Autodesk Inventor part; units mm, degrees
(part 2 of 6)
  line L925 (26.7951, -12.8841) -> (26.6059, -12.8584)
  line L926 (26.6059, -12.8584) -> (26.4288, -12.8305)
  line L927 (26.4288, -12.8305) -> (26.0833, -12.7672)
  line L928 (26.0833, -12.7672) -> (26.0365, -12.7656)
  line L929 (26.0365, -12.7656) -> (26.0012, -12.7712)
  line L930 (26.0012, -12.7712) -> (25.9777, -12.7837)
  line L931 (25.9777, -12.7837) -> (25.968, -12.7973)
  line L932 (25.968, -12.7973) -> (25.7946, -13.143)
  line L933 (25.7946, -13.143) -> (25.6168, -13.4865)
  line L934 (25.6168, -13.4865) -> (25.6116, -13.5023)
  line L935 (25.6116, -13.5023) -> (25.6153, -13.5287)
  line L936 (25.6153, -13.5287) -> (25.6314, -13.5605)
  line L937 (25.6314, -13.5605) -> (25.6603, -13.5974)
  line L938 (25.6603, -13.5974) -> (25.9146, -13.8398)
  line L939 (25.9146, -13.8398) -> (26.0412, -13.9666)
  line L940 (26.0412, -13.9666) -> (26.1732, -14.1046)
  line L941 (26.1732, -14.1046) -> (26.312, -14.2558)
  line L942 (26.312, -14.2558) -> (26.455, -14.4184)
  line L943 (26.455, -14.4184) -> (26.602, -14.5927)
  line L944 (26.602, -14.5927) -> (26.7541, -14.7808)
  line L945 (26.7541, -14.7808) -> (26.9091, -14.9811)
  line L946 (26.9091, -14.9811) -> (27.041, -15.1586)
  arc A24 (26.6482, -15.8389) -> (27.041, -15.1586) centre (0, 0) ccw
  line L947 (26.6482, -15.8389) -> (26.4285, -15.8134)
  line L948 (26.4285, -15.8134) -> (26.1776, -15.7793)
  line L949 (26.1776, -15.7793) -> (25.9387, -15.7417)
  line L950 (25.9387, -15.7417) -> (25.7142, -15.7015)
  line L951 (25.7142, -15.7015) -> (25.5018, -15.6589)
  line L952 (25.5018, -15.6589) -> (25.3015, -15.6144)
  line L953 (25.3015, -15.6144) -> (25.1161, -15.569)
  line L954 (25.1161, -15.569) -> (24.9429, -15.5228)
  line L955 (24.9429, -15.5228) -> (24.6058, -15.4237)
  line L956 (24.6058, -15.4237) -> (24.5595, -15.4172)
  line L957 (24.5595, -15.4172) -> (24.5238, -15.4191)
  line L958 (24.5238, -15.4191) -> (24.4991, -15.4291)
  line L959 (24.4991, -15.4291) -> (24.488, -15.4416)
  line L960 (24.488, -15.4416) -> (24.2795, -15.7673)
  line L961 (24.2795, -15.7673) -> (24.0668, -16.0903)
  line L962 (24.0668, -16.0903) -> (24.0599, -16.1055)
  line L963 (24.0599, -16.1055) -> (24.0608, -16.1321)
  line L964 (24.0608, -16.1321) -> (24.0735, -16.1655)
  line L965 (24.0735, -16.1655) -> (24.0984, -16.2052)
  line L966 (24.0984, -16.2052) -> (24.326, -16.4728)
  line L967 (24.326, -16.4728) -> (24.4386, -16.6122)
  line L968 (24.4386, -16.6122) -> (24.5555, -16.7632)
  line L969 (24.5555, -16.7632) -> (24.6777, -16.928)
  line L970 (24.6777, -16.928) -> (24.8029, -17.1047)
  line L971 (24.8029, -17.1047) -> (24.931, -17.2934)
  line L972 (24.931, -17.2934) -> (25.0625, -17.4964)
  line L973 (25.0625, -17.4964) -> (25.1957, -17.7118)
  line L974 (25.1957, -17.7118) -> (25.3084, -17.9021)
  arc A25 (24.8466, -18.5377) -> (25.3084, -17.9021) centre (0, 0) ccw
  line L975 (24.8466, -18.5377) -> (24.6308, -18.4893)
  line L976 (24.6308, -18.4893) -> (24.3848, -18.4292)
  line L977 (24.3848, -18.4292) -> (24.1511, -18.3668)
  line L978 (24.1511, -18.3668) -> (23.932, -18.3034)
  line L979 (23.932, -18.3034) -> (23.7253, -18.2388)
  line L980 (23.7253, -18.2388) -> (23.5308, -18.1736)
  line L981 (23.5308, -18.1736) -> (23.3511, -18.1091)
  line L982 (23.3511, -18.1091) -> (23.1837, -18.045)
  line L983 (23.1837, -18.045) -> (22.8588, -17.9112)
  line L984 (22.8588, -17.9112) -> (22.8134, -17.8999)
  line L985 (22.8134, -17.8999) -> (22.7777, -17.8981)
  line L986 (22.7777, -17.8981) -> (22.7521, -17.9055)
  line L987 (22.7521, -17.9055) -> (22.7398, -17.9167)
  line L988 (22.7398, -17.9167) -> (22.4984, -18.2188)
  line L989 (22.4984, -18.2188) -> (22.2531, -18.5178)
  line L990 (22.2531, -18.5178) -> (22.2446, -18.5322)
  line L991 (22.2446, -18.5322) -> (22.2427, -18.5587)
  line L992 (22.2427, -18.5587) -> (22.2519, -18.5933)
  line L993 (22.2519, -18.5933) -> (22.2724, -18.6353)
  line L994 (22.2724, -18.6353) -> (22.4708, -18.9253)
  line L995 (22.4708, -18.9253) -> (22.5683, -19.0757)
  line L996 (22.5683, -19.0757) -> (22.6688, -19.2381)
  line L997 (22.6688, -19.2381) -> (22.773, -19.4148)
  line L998 (22.773, -19.4148) -> (22.8791, -19.6036)
  line L999 (22.8791, -19.6036) -> (22.9867, -19.8047)
  line L1000 (22.9867, -19.8047) -> (23.0963, -20.0203)
  line L1001 (23.0963, -20.0203) -> (23.2063, -20.2484)
  line L1002 (23.2063, -20.2484) -> (23.2985, -20.4495)
  arc A26 (22.7728, -21.0333) -> (23.2985, -20.4495) centre (0, 0) ccw
  line L1003 (22.7728, -21.0333) -> (22.5632, -20.9626)
  line L1004 (22.5632, -20.9626) -> (22.3249, -20.8771)
  line L1005 (22.3249, -20.8771) -> (22.099, -20.7906)
  line L1006 (22.099, -20.7906) -> (21.8877, -20.7047)
  line L1007 (21.8877, -20.7047) -> (21.6889, -20.6189)
  line L1008 (21.6889, -20.6189) -> (21.5022, -20.5336)
  line L1009 (21.5022, -20.5336) -> (21.3302, -20.4507)
  line L1010 (21.3302, -20.4507) -> (21.1705, -20.3695)
  line L1011 (21.1705, -20.3695) -> (20.8614, -20.2025)
  line L1012 (20.8614, -20.2025) -> (20.8174, -20.1865)
  line L1013 (20.8174, -20.1865) -> (20.7821, -20.181)
  line L1014 (20.7821, -20.181) -> (20.7559, -20.1856)
  line L1015 (20.7559, -20.1856) -> (20.7424, -20.1955)
  line L1016 (20.7424, -20.1955) -> (20.4707, -20.4707)
  line L1017 (20.4707, -20.4707) -> (20.1955, -20.7424)
  line L1018 (20.1955, -20.7424) -> (20.1856, -20.7559)
  line L1019 (20.1856, -20.7559) -> (20.181, -20.7821)
  line L1020 (20.181, -20.7821) -> (20.1865, -20.8174)
  line L1021 (20.1865, -20.8174) -> (20.2025, -20.8614)
  line L1022 (20.2025, -20.8614) -> (20.3695, -21.1705)
  line L1023 (20.3695, -21.1705) -> (20.4507, -21.3302)
  line L1024 (20.4507, -21.3302) -> (20.5336, -21.5022)
  line L1025 (20.5336, -21.5022) -> (20.6189, -21.6889)
  line L1026 (20.6189, -21.6889) -> (20.7047, -21.8877)
  line L1027 (20.7047, -21.8877) -> (20.7906, -22.099)
  line L1028 (20.7906, -22.099) -> (20.8771, -22.3249)
  line L1029 (20.8771, -22.3249) -> (20.9626, -22.5632)
  line L1030 (20.9626, -22.5632) -> (21.0333, -22.7728)
  arc A27 (20.4495, -23.2985) -> (21.0333, -22.7728) centre (0, 0) ccw
  line L1031 (20.4495, -23.2985) -> (20.2484, -23.2063)
  line L1032 (20.2484, -23.2063) -> (20.0203, -23.0963)
  line L1033 (20.0203, -23.0963) -> (19.8047, -22.9867)
  line L1034 (19.8047, -22.9867) -> (19.6036, -22.8791)
  line L1035 (19.6036, -22.8791) -> (19.4148, -22.773)
  line L1036 (19.4148, -22.773) -> (19.2381, -22.6688)
  line L1037 (19.2381, -22.6688) -> (19.0757, -22.5683)
  line L1038 (19.0757, -22.5683) -> (18.9253, -22.4708)
  line L1039 (18.9253, -22.4708) -> (18.6353, -22.2724)
  line L1040 (18.6353, -22.2724) -> (18.5933, -22.2519)
  line L1041 (18.5933, -22.2519) -> (18.5587, -22.2427)
  line L1042 (18.5587, -22.2427) -> (18.5322, -22.2446)
  line L1043 (18.5322, -22.2446) -> (18.5178, -22.2531)
  line L1044 (18.5178, -22.2531) -> (18.2188, -22.4984)
  line L1045 (18.2188, -22.4984) -> (17.9167, -22.7398)
  line L1046 (17.9167, -22.7398) -> (17.9055, -22.7521)
  line L1047 (17.9055, -22.7521) -> (17.8981, -22.7777)
  line L1048 (17.8981, -22.7777) -> (17.8999, -22.8134)
  line L1049 (17.8999, -22.8134) -> (17.9112, -22.8588)
  line L1050 (17.9112, -22.8588) -> (18.045, -23.1837)
  line L1051 (18.045, -23.1837) -> (18.1091, -23.3511)
  line L1052 (18.1091, -23.3511) -> (18.1736, -23.5308)
  line L1053 (18.1736, -23.5308) -> (18.2388, -23.7253)
  line L1054 (18.2388, -23.7253) -> (18.3034, -23.932)
  line L1055 (18.3034, -23.932) -> (18.3668, -24.1511)
  line L1056 (18.3668, -24.1511) -> (18.4292, -24.3848)
  line L1057 (18.4292, -24.3848) -> (18.4893, -24.6308)
  line L1058 (18.4893, -24.6308) -> (18.5377, -24.8466)
  arc A28 (17.9021, -25.3084) -> (18.5377, -24.8466) centre (0, 0) ccw
  line L1059 (17.9021, -25.3084) -> (17.7118, -25.1957)
  line L1060 (17.7118, -25.1957) -> (17.4964, -25.0625)
  line L1061 (17.4964, -25.0625) -> (17.2934, -24.931)
  line L1062 (17.2934, -24.931) -> (17.1047, -24.8029)
  line L1063 (17.1047, -24.8029) -> (16.928, -24.6777)
  line L1064 (16.928, -24.6777) -> (16.7632, -24.5555)
  line L1065 (16.7632, -24.5555) -> (16.6122, -24.4386)
  line L1066 (16.6122, -24.4386) -> (16.4728, -24.326)
  line L1067 (16.4728, -24.326) -> (16.2052, -24.0984)
  line L1068 (16.2052, -24.0984) -> (16.1655, -24.0735)
  line L1069 (16.1655, -24.0735) -> (16.1321, -24.0608)
  line L1070 (16.1321, -24.0608) -> (16.1055, -24.0599)
  line L1071 (16.1055, -24.0599) -> (16.0903, -24.0668)
  line L1072 (16.0903, -24.0668) -> (15.7673, -24.2795)
  line L1073 (15.7673, -24.2795) -> (15.4416, -24.488)
  line L1074 (15.4416, -24.488) -> (15.4291, -24.4991)
  line L1075 (15.4291, -24.4991) -> (15.4191, -24.5238)
  line L1076 (15.4191, -24.5238) -> (15.4172, -24.5595)
  line L1077 (15.4172, -24.5595) -> (15.4237, -24.6058)
  line L1078 (15.4237, -24.6058) -> (15.5228, -24.9429)
  line L1079 (15.5228, -24.9429) -> (15.569, -25.1161)
  line L1080 (15.569, -25.1161) -> (15.6144, -25.3015)
  line L1081 (15.6144, -25.3015) -> (15.6589, -25.5018)
  line L1082 (15.6589, -25.5018) -> (15.7015, -25.7142)
  line L1083 (15.7015, -25.7142) -> (15.7417, -25.9387)
  line L1084 (15.7417, -25.9387) -> (15.7793, -26.1776)
  line L1085 (15.7793, -26.1776) -> (15.8134, -26.4285)
  line L1086 (15.8134, -26.4285) -> (15.8389, -26.6482)
  arc A29 (15.1586, -27.041) -> (15.8389, -26.6482) centre (0, 0) ccw
  line L1087 (15.1586, -27.041) -> (14.9811, -26.9091)
  line L1088 (14.9811, -26.9091) -> (14.7808, -26.7541)
  line L1089 (14.7808, -26.7541) -> (14.5927, -26.602)
  line L1090 (14.5927, -26.602) -> (14.4184, -26.455)
  line L1091 (14.4184, -26.455) -> (14.2558, -26.312)
  line L1092 (14.2558, -26.312) -> (14.1046, -26.1732)
  line L1093 (14.1046, -26.1732) -> (13.9666, -26.0412)
  line L1094 (13.9666, -26.0412) -> (13.8398, -25.9146)
  line L1095 (13.8398, -25.9146) -> (13.5974, -25.6603)
  line L1096 (13.5974, -25.6603) -> (13.5605, -25.6314)
  line L1097 (13.5605, -25.6314) -> (13.5287, -25.6153)
  line L1098 (13.5287, -25.6153) -> (13.5023, -25.6116)
  line L1099 (13.5023, -25.6116) -> (13.4865, -25.6168)
  line L1100 (13.4865, -25.6168) -> (13.143, -25.7946)
  line L1101 (13.143, -25.7946) -> (12.7973, -25.968)
  line L1102 (12.7973, -25.968) -> (12.7837, -25.9777)
  line L1103 (12.7837, -25.9777) -> (12.7712, -26.0012)
  line L1104 (12.7712, -26.0012) -> (12.7656, -26.0365)
  line L1105 (12.7656, -26.0365) -> (12.7672, -26.0833)
  line L1106 (12.7672, -26.0833) -> (12.8305, -26.4288)
  line L1107 (12.8305, -26.4288) -> (12.8584, -26.6059)
  line L1108 (12.8584, -26.6059) -> (12.8841, -26.7951)
  line L1109 (12.8841, -26.7951) -> (12.9075, -26.9989)
  line L1110 (12.9075, -26.9989) -> (12.9276, -27.2145)
  line L1111 (12.9276, -27.2145) -> (12.9441, -27.442)
  line L1112 (12.9441, -27.442) -> (12.9565, -27.6836)
  line L1113 (12.9565, -27.6836) -> (12.9642, -27.9367)
  line L1114 (12.9642, -27.9367) -> (12.9667, -28.1579)
  arc A30 (12.249, -28.4774) -> (12.9667, -28.1579) centre (0, 0) ccw
  line L1115 (12.249, -28.4774) -> (12.0862, -28.3276)
  line L1116 (12.0862, -28.3276) -> (11.9033, -28.1525)
  line L1117 (11.9033, -28.1525) -> (11.7321, -27.9817)
  line L1118 (11.7321, -27.9817) -> (11.5741, -27.8172)
  line L1119 (11.5741, -27.8172) -> (11.4273, -27.6579)
  line L1120 (11.4273, -27.6579) -> (11.2915, -27.5042)
  line L1121 (11.2915, -27.5042) -> (11.1681, -27.3584)
  line L1122 (11.1681, -27.3584) -> (11.0551, -27.2193)
  line L1123 (11.0551, -27.2193) -> (10.8407, -26.941)
  line L1124 (10.8407, -26.941) -> (10.807, -26.9085)
  line L1125 (10.807, -26.9085) -> (10.777, -26.8891)
  line L1126 (10.777, -26.8891) -> (10.7512, -26.8826)
  line L1127 (10.7512, -26.8826) -> (10.7349, -26.8862)
  line L1128 (10.7349, -26.8862) -> (10.3748, -27.0272)
  line L1129 (10.3748, -27.0272) -> (10.0128, -27.1634)
  line L1130 (10.0128, -27.1634) -> (9.9983, -27.1717)
  line L1131 (9.9983, -27.1717) -> (9.9834, -27.1937)
  line L1132 (9.9834, -27.1937) -> (9.9741, -27.2282)
  line L1133 (9.9741, -27.2282) -> (9.9708, -27.2749)
  line L1134 (9.9708, -27.2749) -> (9.9977, -27.6252)
  line L1135 (9.9977, -27.6252) -> (10.0069, -27.8042)
  line L1136 (10.0069, -27.8042) -> (10.0127, -27.995)
  line L1137 (10.0127, -27.995) -> (10.0146, -28.2002)
  line L1138 (10.0146, -28.2002) -> (10.0121, -28.4168)
  line L1139 (10.0121, -28.4168) -> (10.0047, -28.6447)
  line L1140 (10.0047, -28.6447) -> (9.9918, -28.8863)
  line L1141 (9.9918, -28.8863) -> (9.973, -29.1388)
  line L1142 (9.973, -29.1388) -> (9.9523, -29.359)
  arc A31 (9.2052, -29.6018) -> (9.9523, -29.359) centre (0, 0) ccw
  line L1143 (9.2052, -29.6018) -> (9.059, -29.4358)
  line L1144 (9.059, -29.4358) -> (8.8954, -29.2425)
  line L1145 (8.8954, -29.2425) -> (8.7429, -29.0547)
  line L1146 (8.7429, -29.0547) -> (8.603, -28.8746)
  line L1147 (8.603, -28.8746) -> (8.4737, -28.7009)
  line L1148 (8.4737, -28.7009) -> (8.3547, -28.5338)
  line L1149 (8.3547, -28.5338) -> (8.2472, -28.3759)
  line L1150 (8.2472, -28.3759) -> (8.1494, -28.2257)
  line L1151 (8.1494, -28.2257) -> (7.9652, -27.9266)
  line L1152 (7.9652, -27.9266) -> (7.9351, -27.8907)
  line L1153 (7.9351, -27.8907) -> (7.9073, -27.8683)
  line L1154 (7.9073, -27.8683) -> (7.8823, -27.8592)
  line L1155 (7.8823, -27.8592) -> (7.8657, -27.861)
  line L1156 (7.8657, -27.861) -> (7.4928, -27.9636)
  line L1157 (7.4928, -27.9636) -> (7.1186, -28.0612)
  line L1158 (7.1186, -28.0612) -> (7.1033, -28.0679)
  line L1159 (7.1033, -28.0679) -> (7.0862, -28.0883)
  line L1160 (7.0862, -28.0883) -> (7.0733, -28.1216)
  line L1161 (7.0733, -28.1216) -> (7.0652, -28.1677)
  line L1162 (7.0652, -28.1677) -> (7.0553, -28.5189)
  line L1163 (7.0553, -28.5189) -> (7.0457, -28.6979)
  line L1164 (7.0457, -28.6979) -> (7.0315, -28.8883)
  line L1165 (7.0315, -28.8883) -> (7.012, -29.0926)
  line L1166 (7.012, -29.0926) -> (6.9869, -29.3077)
  line L1167 (6.9869, -29.3077) -> (6.9557, -29.5336)
  line L1168 (6.9557, -29.5336) -> (6.9177, -29.7725)
  line L1169 (6.9177, -29.7725) -> (6.8726, -30.0216)
  line L1170 (6.8726, -30.0216) -> (6.829, -30.2385)
  arc A32 (6.0605, -30.4018) -> (6.829, -30.2385) centre (0, 0) ccw
  line L1171 (6.0605, -30.4018) -> (5.9325, -30.2214)
  line L1172 (5.9325, -30.2214) -> (5.79, -30.0122)
  line L1173 (5.79, -30.0122) -> (5.658, -29.8094)
  line L1174 (5.658, -29.8094) -> (5.5376, -29.6157)
  line L1175 (5.5376, -29.6157) -> (5.4272, -29.4294)
  line L1176 (5.4272, -29.4294) -> (5.3263, -29.2508)
  line L1177 (5.3263, -29.2508) -> (5.2359, -29.0826)
  line L1178 (5.2359, -29.0826) -> (5.1544, -28.9229)
  line L1179 (5.1544, -28.9229) -> (5.0025, -28.6062)
  line L1180 (5.0025, -28.6062) -> (4.9763, -28.5674)
  line L1181 (4.9763, -28.5674) -> (4.951, -28.5421)
  line L1182 (4.951, -28.5421) -> (4.927, -28.5305)
  line L1183 (4.927, -28.5305) -> (4.9104, -28.5306)
  line L1184 (4.9104, -28.5306) -> (4.5288, -28.5936)
  line L1185 (4.5288, -28.5936) -> (4.1464, -28.6516)
  line L1186 (4.1464, -28.6516) -> (4.1305, -28.6567)
  line L1187 (4.1305, -28.6567) -> (4.1114, -28.6751)
  line L1188 (4.1114, -28.6751) -> (4.0951, -28.7069)
  line L1189 (4.0951, -28.7069) -> (4.0822, -28.7519)
  line L1190 (4.0822, -28.7519) -> (4.0356, -29.1001)
  line L1191 (4.0356, -29.1001) -> (4.0074, -29.2771)
  line L1192 (4.0074, -29.2771) -> (3.9734, -29.465)
  line L1193 (3.9734, -29.465) -> (3.9326, -29.6661)
  line L1194 (3.9326, -29.6661) -> (3.8852, -29.8774)
  line L1195 (3.8852, -29.8774) -> (3.8305, -30.0989)
  line L1196 (3.8305, -30.0989) -> (3.7677, -30.3325)
  line L1197 (3.7677, -30.3325) -> (3.6968, -30.5755)
  line L1198 (3.6968, -30.5755) -> (3.6308, -30.7866)
  arc A33 (2.8495, -30.8688) -> (3.6308, -30.7866) centre (0, 0) ccw
  line L1199 (2.8495, -30.8688) -> (2.741, -30.676)
  line L1200 (2.741, -30.676) -> (2.6211, -30.453)
  line L1201 (2.6211, -30.453) -> (2.5111, -30.2376)
  line L1202 (2.5111, -30.2376) -> (2.4116, -30.0323)
  line L1203 (2.4116, -30.0323) -> (2.3213, -29.8355)
  line L1204 (2.3213, -29.8355) -> (2.2396, -29.6473)
  line L1205 (2.2396, -29.6473) -> (2.1673, -29.4705)
  line L1206 (2.1673, -29.4705) -> (2.1029, -29.3033)
  line L1207 (2.1029, -29.3033) -> (1.9849, -28.9724)
  line L1208 (1.9849, -28.9724) -> (1.9629, -28.931)
  line L1209 (1.9629, -28.931) -> (1.9404, -28.9033)
  line L1210 (1.9404, -28.9033) -> (1.9178, -28.8892)
  line L1211 (1.9178, -28.8892) -> (1.9012, -28.8876)
  line L1212 (1.9012, -28.8876) -> (1.5151, -28.9103)
  line L1213 (1.5151, -28.9103) -> (1.1288, -28.9281)
  line L1214 (1.1288, -28.9281) -> (1.1124, -28.9314)
  line L1215 (1.1124, -28.9314) -> (1.0915, -28.9478)
  line L1216 (1.0915, -28.9478) -> (1.0719, -28.9777)
  line L1217 (1.0719, -28.9777) -> (1.0544, -29.0211)
  line L1218 (1.0544, -29.0211) -> (0.9717, -29.3626)
  line L1219 (0.9717, -29.3626) -> (0.9251, -29.5356)
  line L1220 (0.9251, -29.5356) -> (0.8717, -29.719)
  line L1221 (0.8717, -29.719) -> (0.8101, -29.9147)
  line L1222 (0.8101, -29.9147) -> (0.7408, -30.1199)
  line L1223 (0.7408, -30.1199) -> (0.6634, -30.3344)
  line L1224 (0.6634, -30.3344) -> (0.5765, -30.5601)
  line L1225 (0.5765, -30.5601) -> (0.4805, -30.7945)
  line L1226 (0.4805, -30.7945) -> (0.3928, -30.9975)
  arc A34 (-0.3928, -30.9975) -> (0.3928, -30.9975) centre (0, 0) ccw
  line L1227 (-0.3928, -30.9975) -> (-0.4805, -30.7945)
  line L1228 (-0.4805, -30.7945) -> (-0.5765, -30.5601)
  line L1229 (-0.5765, -30.5601) -> (-0.6634, -30.3344)
  line L1230 (-0.6634, -30.3344) -> (-0.7408, -30.1199)
  line L1231 (-0.7408, -30.1199) -> (-0.8101, -29.9147)
  line L1232 (-0.8101, -29.9147) -> (-0.8717, -29.719)
  line L1233 (-0.8717, -29.719) -> (-0.9251, -29.5356)
  line L1234 (-0.9251, -29.5356) -> (-0.9717, -29.3626)
  line L1235 (-0.9717, -29.3626) -> (-1.0544, -29.0211)
  line L1236 (-1.0544, -29.0211) -> (-1.0719, -28.9777)
  line L1237 (-1.0719, -28.9777) -> (-1.0915, -28.9478)
  line L1238 (-1.0915, -28.9478) -> (-1.1124, -28.9314)
  line L1239 (-1.1124, -28.9314) -> (-1.1288, -28.9281)
  line L1240 (-1.1288, -28.9281) -> (-1.5151, -28.9103)
  line L1241 (-1.5151, -28.9103) -> (-1.9012, -28.8876)
  line L1242 (-1.9012, -28.8876) -> (-1.9178, -28.8892)
  line L1243 (-1.9178, -28.8892) -> (-1.9404, -28.9033)
  line L1244 (-1.9404, -28.9033) -> (-1.9629, -28.931)
  line L1245 (-1.9629, -28.931) -> (-1.9849, -28.9724)
  line L1246 (-1.9849, -28.9724) -> (-2.1029, -29.3033)
  line L1247 (-2.1029, -29.3033) -> (-2.1673, -29.4705)
  line L1248 (-2.1673, -29.4705) -> (-2.2396, -29.6473)
  line L1249 (-2.2396, -29.6473) -> (-2.3213, -29.8355)
  line L1250 (-2.3213, -29.8355) -> (-2.4116, -30.0323)
  line L1251 (-2.4116, -30.0323) -> (-2.5111, -30.2376)
  line L1252 (-2.5111, -30.2376) -> (-2.6211, -30.453)
  line L1253 (-2.6211, -30.453) -> (-2.741, -30.676)
  line L1254 (-2.741, -30.676) -> (-2.8495, -30.8688)
  arc A35 (-3.6308, -30.7866) -> (-2.8495, -30.8688) centre (0, 0) ccw
  line L1255 (-3.6308, -30.7866) -> (-3.6968, -30.5755)
  line L1256 (-3.6968, -30.5755) -> (-3.7677, -30.3325)
  line L1257 (-3.7677, -30.3325) -> (-3.8305, -30.0989)
  line L1258 (-3.8305, -30.0989) -> (-3.8852, -29.8774)
  line L1259 (-3.8852, -29.8774) -> (-3.9326, -29.6661)
  line L1260 (-3.9326, -29.6661) -> (-3.9734, -29.465)
  line L1261 (-3.9734, -29.465) -> (-4.0074, -29.2771)
  line L1262 (-4.0074, -29.2771) -> (-4.0356, -29.1001)
  line L1263 (-4.0356, -29.1001) -> (-4.0822, -28.7519)
  line L1264 (-4.0822, -28.7519) -> (-4.0951, -28.7069)
  line L1265 (-4.0951, -28.7069) -> (-4.1114, -28.6751)
  line L1266 (-4.1114, -28.6751) -> (-4.1305, -28.6567)
  line L1267 (-4.1305, -28.6567) -> (-4.1464, -28.6516)
  line L1268 (-4.1464, -28.6516) -> (-4.5288, -28.5936)
  line L1269 (-4.5288, -28.5936) -> (-4.9104, -28.5306)
  line L1270 (-4.9104, -28.5306) -> (-4.927, -28.5305)
  line L1271 (-4.927, -28.5305) -> (-4.951, -28.5421)
  line L1272 (-4.951, -28.5421) -> (-4.9763, -28.5674)
  line L1273 (-4.9763, -28.5674) -> (-5.0025, -28.6062)
  line L1274 (-5.0025, -28.6062) -> (-5.1544, -28.9229)
  line L1275 (-5.1544, -28.9229) -> (-5.2359, -29.0826)
  line L1276 (-5.2359, -29.0826) -> (-5.3263, -29.2508)
  line L1277 (-5.3263, -29.2508) -> (-5.4272, -29.4294)
  line L1278 (-5.4272, -29.4294) -> (-5.5376, -29.6157)
  line L1279 (-5.5376, -29.6157) -> (-5.658, -29.8094)
  line L1280 (-5.658, -29.8094) -> (-5.79, -30.0122)
  line L1281 (-5.79, -30.0122) -> (-5.9325, -30.2214)
  line L1282 (-5.9325, -30.2214) -> (-6.0605, -30.4018)
  arc A36 (-6.829, -30.2385) -> (-6.0605, -30.4018) centre (0, 0) ccw
  line L1283 (-6.829, -30.2385) -> (-6.8726, -30.0216)
  line L1284 (-6.8726, -30.0216) -> (-6.9177, -29.7725)
  line L1285 (-6.9177, -29.7725) -> (-6.9557, -29.5336)
  line L1286 (-6.9557, -29.5336) -> (-6.9869, -29.3077)
  line L1287 (-6.9869, -29.3077) -> (-7.012, -29.0926)
  line L1288 (-7.012, -29.0926) -> (-7.0315, -28.8883)
  line L1289 (-7.0315, -28.8883) -> (-7.0457, -28.6979)
  line L1290 (-7.0457, -28.6979) -> (-7.0553, -28.5189)
  line L1291 (-7.0553, -28.5189) -> (-7.0652, -28.1677)
  line L1292 (-7.0652, -28.1677) -> (-7.0733, -28.1216)
  line L1293 (-7.0733, -28.1216) -> (-7.0862, -28.0883)
  line L1294 (-7.0862, -28.0883) -> (-7.1033, -28.0679)
  line L1295 (-7.1033, -28.0679) -> (-7.1186, -28.0612)
  line L1296 (-7.1186, -28.0612) -> (-7.4928, -27.9636)
  line L1297 (-7.4928, -27.9636) -> (-7.8657, -27.861)
  line L1298 (-7.8657, -27.861) -> (-7.8823, -27.8592)
  line L1299 (-7.8823, -27.8592) -> (-7.9073, -27.8683)
  line L1300 (-7.9073, -27.8683) -> (-7.9351, -27.8907)
  line L1301 (-7.9351, -27.8907) -> (-7.9652, -27.9266)
  line L1302 (-7.9652, -27.9266) -> (-8.1494, -28.2257)
  line L1303 (-8.1494, -28.2257) -> (-8.2472, -28.3759)
  line L1304 (-8.2472, -28.3759) -> (-8.3547, -28.5338)
  line L1305 (-8.3547, -28.5338) -> (-8.4737, -28.7009)
  line L1306 (-8.4737, -28.7009) -> (-8.603, -28.8746)
  line L1307 (-8.603, -28.8746) -> (-8.7429, -29.0547)
  line L1308 (-8.7429, -29.0547) -> (-8.8954, -29.2425)
  line L1309 (-8.8954, -29.2425) -> (-9.059, -29.4358)
  line L1310 (-9.059, -29.4358) -> (-9.2052, -29.6018)
  arc A37 (-9.9523, -29.359) -> (-9.2052, -29.6018) centre (0, 0) ccw
  line L1311 (-9.9523, -29.359) -> (-9.973, -29.1388)
  line L1312 (-9.973, -29.1388) -> (-9.9918, -28.8863)
  line L1313 (-9.9918, -28.8863) -> (-10.0047, -28.6447)
  line L1314 (-10.0047, -28.6447) -> (-10.0121, -28.4168)
  line L1315 (-10.0121, -28.4168) -> (-10.0146, -28.2002)
  line L1316 (-10.0146, -28.2002) -> (-10.0127, -27.995)
  line L1317 (-10.0127, -27.995) -> (-10.0069, -27.8042)
  line L1318 (-10.0069, -27.8042) -> (-9.9977, -27.6252)
  line L1319 (-9.9977, -27.6252) -> (-9.9708, -27.2749)
  line L1320 (-9.9708, -27.2749) -> (-9.9741, -27.2282)
  line L1321 (-9.9741, -27.2282) -> (-9.9834, -27.1937)
  line L1322 (-9.9834, -27.1937) -> (-9.9983, -27.1717)
  line L1323 (-9.9983, -27.1717) -> (-10.0128, -27.1634)
  line L1324 (-10.0128, -27.1634) -> (-10.3748, -27.0272)
  line L1325 (-10.3748, -27.0272) -> (-10.7349, -26.8862)
  line L1326 (-10.7349, -26.8862) -> (-10.7512, -26.8826)
  line L1327 (-10.7512, -26.8826) -> (-10.777, -26.8891)
  line L1328 (-10.777, -26.8891) -> (-10.807, -26.9085)
  line L1329 (-10.807, -26.9085) -> (-10.8407, -26.941)
  line L1330 (-10.8407, -26.941) -> (-11.0551, -27.2193)
  line L1331 (-11.0551, -27.2193) -> (-11.1681, -27.3584)
  line L1332 (-11.1681, -27.3584) -> (-11.2915, -27.5042)
  line L1333 (-11.2915, -27.5042) -> (-11.4273, -27.6579)
  line L1334 (-11.4273, -27.6579) -> (-11.5741, -27.8172)
  line L1335 (-11.5741, -27.8172) -> (-11.7321, -27.9817)
  line L1336 (-11.7321, -27.9817) -> (-11.9033, -28.1525)
  line L1337 (-11.9033, -28.1525) -> (-12.0862, -28.3276)
  line L1338 (-12.0862, -28.3276) -> (-12.249, -28.4774)
  arc A38 (-12.9667, -28.1579) -> (-12.249, -28.4774) centre (0, 0) ccw
  line L1339 (-12.9667, -28.1579) -> (-12.9642, -27.9367)
  line L1340 (-12.9642, -27.9367) -> (-12.9565, -27.6836)
  line L1341 (-12.9565, -27.6836) -> (-12.9441, -27.442)
  line L1342 (-12.9441, -27.442) -> (-12.9276, -27.2145)
  line L1343 (-12.9276, -27.2145) -> (-12.9075, -26.9989)
  line L1344 (-12.9075, -26.9989) -> (-12.8841, -26.7951)
  line L1345 (-12.8841, -26.7951) -> (-12.8584, -26.6059)
  line L1346 (-12.8584, -26.6059) -> (-12.8305, -26.4288)
  line L1347 (-12.8305, -26.4288) -> (-12.7672, -26.0833)
  line L1348 (-12.7672, -26.0833) -> (-12.7656, -26.0365)
  line L1349 (-12.7656, -26.0365) -> (-12.7712, -26.0012)
  line L1350 (-12.7712, -26.0012) -> (-12.7837, -25.9777)
  line L1351 (-12.7837, -25.9777) -> (-12.7973, -25.968)
  line L1352 (-12.7973, -25.968) -> (-13.143, -25.7946)
  line L1353 (-13.143, -25.7946) -> (-13.4865, -25.6168)
  line L1354 (-13.4865, -25.6168) -> (-13.5023, -25.6116)
  line L1355 (-13.5023, -25.6116) -> (-13.5287, -25.6153)
  line L1356 (-13.5287, -25.6153) -> (-13.5605, -25.6314)
  line L1357 (-13.5605, -25.6314) -> (-13.5974, -25.6603)
  line L1358 (-13.5974, -25.6603) -> (-13.8398, -25.9146)
  line L1359 (-13.8398, -25.9146) -> (-13.9666, -26.0412)
  line L1360 (-13.9666, -26.0412) -> (-14.1046, -26.1732)
  line L1361 (-14.1046, -26.1732) -> (-14.2558, -26.312)
  line L1362 (-14.2558, -26.312) -> (-14.4184, -26.455)
  line L1363 (-14.4184, -26.455) -> (-14.5927, -26.602)
  line L1364 (-14.5927, -26.602) -> (-14.7808, -26.7541)
  line L1365 (-14.7808, -26.7541) -> (-14.9811, -26.9091)
  line L1366 (-14.9811, -26.9091) -> (-15.1586, -27.041)
  arc A39 (-15.8389, -26.6482) -> (-15.1586, -27.041) centre (0, 0) ccw
  line L1367 (-15.8389, -26.6482) -> (-15.8134, -26.4285)
  line L1368 (-15.8134, -26.4285) -> (-15.7793, -26.1776)
  line L1369 (-15.7793, -26.1776) -> (-15.7417, -25.9387)
  line L1370 (-15.7417, -25.9387) -> (-15.7015, -25.7142)
  line L1371 (-15.7015, -25.7142) -> (-15.6589, -25.5018)
  line L1372 (-15.6589, -25.5018) -> (-15.6144, -25.3015)
  line L1373 (-15.6144, -25.3015) -> (-15.569, -25.1161)
  line L1374 (-15.569, -25.1161) -> (-15.5228, -24.9429)
  line L1375 (-15.5228, -24.9429) -> (-15.4237, -24.6058)
  line L1376 (-15.4237, -24.6058) -> (-15.4172, -24.5595)
  line L1377 (-15.4172, -24.5595) -> (-15.4191, -24.5238)
  line L1378 (-15.4191, -24.5238) -> (-15.4291, -24.4991)
  line L1379 (-15.4291, -24.4991) -> (-15.4416, -24.488)
  line L1380 (-15.4416, -24.488) -> (-15.7673, -24.2795)
  line L1381 (-15.7673, -24.2795) -> (-16.0903, -24.0668)
  line L1382 (-16.0903, -24.0668) -> (-16.1055, -24.0599)
  line L1383 (-16.1055, -24.0599) -> (-16.1321, -24.0608)
  line L1384 (-16.1321, -24.0608) -> (-16.1655, -24.0735)
  line L1385 (-16.1655, -24.0735) -> (-16.2052, -24.0984)
  line L1386 (-16.2052, -24.0984) -> (-16.4728, -24.326)
  line L1387 (-16.4728, -24.326) -> (-16.6122, -24.4386)
  line L1388 (-16.6122, -24.4386) -> (-16.7632, -24.5555)
  line L1389 (-16.7632, -24.5555) -> (-16.928, -24.6777)
  line L1390 (-16.928, -24.6777) -> (-17.1047, -24.8029)
  line L1391 (-17.1047, -24.8029) -> (-17.2934, -24.931)
  line L1392 (-17.2934, -24.931) -> (-17.4964, -25.0625)
  line L1393 (-17.4964, -25.0625) -> (-17.7118, -25.1957)
  line L1394 (-17.7118, -25.1957) -> (-17.9021, -25.3084)
  arc A40 (-18.5377, -24.8466) -> (-17.9021, -25.3084) centre (0, 0) ccw
  line L1395 (-18.5377, -24.8466) -> (-18.4893, -24.6308)
  line L1396 (-18.4893, -24.6308) -> (-18.4292, -24.3848)
  line L1397 (-18.4292, -24.3848) -> (-18.3668, -24.1511)
  line L1398 (-18.3668, -24.1511) -> (-18.3034, -23.932)
  line L1399 (-18.3034, -23.932) -> (-18.2388, -23.7253)
  line L1400 (-18.2388, -23.7253) -> (-18.1736, -23.5308)
  line L1401 (-18.1736, -23.5308) -> (-18.1091, -23.3511)
  line L1402 (-18.1091, -23.3511) -> (-18.045, -23.1837)
  line L1403 (-18.045, -23.1837) -> (-17.9112, -22.8588)
  line L1404 (-17.9112, -22.8588) -> (-17.8999, -22.8134)
  line L1405 (-17.8999, -22.8134) -> (-17.8981, -22.7777)
  line L1406 (-17.8981, -22.7777) -> (-17.9055, -22.7521)
  line L1407 (-17.9055, -22.7521) -> (-17.9167, -22.7398)
  line L1408 (-17.9167, -22.7398) -> (-18.2188, -22.4984)
  line L1409 (-18.2188, -22.4984) -> (-18.5178, -22.2531)
  line L1410 (-18.5178, -22.2531) -> (-18.5322, -22.2446)
  line L1411 (-18.5322, -22.2446) -> (-18.5587, -22.2427)
  line L1412 (-18.5587, -22.2427) -> (-18.5933, -22.2519)
  line L1413 (-18.5933, -22.2519) -> (-18.6353, -22.2724)
  line L1414 (-18.6353, -22.2724) -> (-18.9253, -22.4708)
  line L1415 (-18.9253, -22.4708) -> (-19.0757, -22.5683)
  line L1416 (-19.0757, -22.5683) -> (-19.2381, -22.6688)
  line L1417 (-19.2381, -22.6688) -> (-19.4148, -22.773)
  line L1418 (-19.4148, -22.773) -> (-19.6036, -22.8791)
  line L1419 (-19.6036, -22.8791) -> (-19.8047, -22.9867)
  line L1420 (-19.8047, -22.9867) -> (-20.0203, -23.0963)
  line L1421 (-20.0203, -23.0963) -> (-20.2484, -23.2063)
  line L1422 (-20.2484, -23.2063) -> (-20.4495, -23.2985)
  arc A41 (-21.0333, -22.7728) -> (-20.4495, -23.2985) centre (0, 0) ccw
  line L1423 (-21.0333, -22.7728) -> (-20.9626, -22.5632)
  line L1424 (-20.9626, -22.5632) -> (-20.8771, -22.3249)
  line L1425 (-20.8771, -22.3249) -> (-20.7906, -22.099)
  line L1426 (-20.7906, -22.099) -> (-20.7047, -21.8877)
  line L1427 (-20.7047, -21.8877) -> (-20.6189, -21.6889)
  line L1428 (-20.6189, -21.6889) -> (-20.5336, -21.5022)
  line L1429 (-20.5336, -21.5022) -> (-20.4507, -21.3302)
  line L1430 (-20.4507, -21.3302) -> (-20.3695, -21.1705)
  line L1431 (-20.3695, -21.1705) -> (-20.2025, -20.8614)
  line L1432 (-20.2025, -20.8614) -> (-20.1865, -20.8174)
  line L1433 (-20.1865, -20.8174) -> (-20.181, -20.7821)
  line L1434 (-20.181, -20.7821) -> (-20.1856, -20.7559)
  line L1435 (-20.1856, -20.7559) -> (-20.1955, -20.7424)
  line L1436 (-20.1955, -20.7424) -> (-20.4707, -20.4707)
  line L1437 (-20.4707, -20.4707) -> (-20.7424, -20.1955)
  line L1438 (-20.7424, -20.1955) -> (-20.7559, -20.1856)
  line L1439 (-20.7559, -20.1856) -> (-20.7821, -20.181)
  line L1440 (-20.7821, -20.181) -> (-20.8174, -20.1865)
  line L1441 (-20.8174, -20.1865) -> (-20.8614, -20.2025)
  line L1442 (-20.8614, -20.2025) -> (-21.1705, -20.3695)
  line L1443 (-21.1705, -20.3695) -> (-21.3302, -20.4507)
  line L1444 (-21.3302, -20.4507) -> (-21.5022, -20.5336)
  line L1445 (-21.5022, -20.5336) -> (-21.6889, -20.6189)
  line L1446 (-21.6889, -20.6189) -> (-21.8877, -20.7047)
  line L1447 (-21.8877, -20.7047) -> (-22.099, -20.7906)
  line L1448 (-22.099, -20.7906) -> (-22.3249, -20.8771)
  line L1449 (-22.3249, -20.8771) -> (-22.5632, -20.9626)
  line L1450 (-22.5632, -20.9626) -> (-22.7728, -21.0333)
  arc A42 (-23.2985, -20.4495) -> (-22.7728, -21.0333) centre (0, 0) ccw
  line L1451 (-23.2985, -20.4495) -> (-23.2063, -20.2484)
  line L1452 (-23.2063, -20.2484) -> (-23.0963, -20.0203)
  line L1453 (-23.0963, -20.0203) -> (-22.9867, -19.8047)
  line L1454 (-22.9867, -19.8047) -> (-22.8791, -19.6036)
  line L1455 (-22.8791, -19.6036) -> (-22.773, -19.4148)
  line L1456 (-22.773, -19.4148) -> (-22.6688, -19.2381)
  line L1457 (-22.6688, -19.2381) -> (-22.5683, -19.0757)
  line L1458 (-22.5683, -19.0757) -> (-22.4708, -18.9253)
  line L1459 (-22.4708, -18.9253) -> (-22.2724, -18.6353)
  line L1460 (-22.2724, -18.6353) -> (-22.2519, -18.5933)
  line L1461 (-22.2519, -18.5933) -> (-22.2427, -18.5587)
  line L1462 (-22.2427, -18.5587) -> (-22.2446, -18.5322)
  line L1463 (-22.2446, -18.5322) -> (-22.2531, -18.5178)
  line L1464 (-22.2531, -18.5178) -> (-22.4984, -18.2188)
  line L1465 (-22.4984, -18.2188) -> (-22.7398, -17.9167)
  line L1466 (-22.7398, -17.9167) -> (-22.7521, -17.9055)
  line L1467 (-22.7521, -17.9055) -> (-22.7777, -17.8981)
  line L1468 (-22.7777, -17.8981) -> (-22.8134, -17.8999)
  line L1469 (-22.8134, -17.8999) -> (-22.8588, -17.9112)
  line L1470 (-22.8588, -17.9112) -> (-23.1837, -18.045)
  line L1471 (-23.1837, -18.045) -> (-23.3511, -18.1091)
  line L1472 (-23.3511, -18.1091) -> (-23.5308, -18.1736)
  line L1473 (-23.5308, -18.1736) -> (-23.7253, -18.2388)
  line L1474 (-23.7253, -18.2388) -> (-23.932, -18.3034)
  line L1475 (-23.932, -18.3034) -> (-24.1511, -18.3668)
  line L1476 (-24.1511, -18.3668) -> (-24.3848, -18.4292)
  line L1477 (-24.3848, -18.4292) -> (-24.6308, -18.4893)
  line L1478 (-24.6308, -18.4893) -> (-24.8466, -18.5377)
  arc A43 (-25.3084, -17.9021) -> (-24.8466, -18.5377) centre (0, 0) ccw
  line L1479 (-25.3084, -17.9021) -> (-25.1957, -17.7118)
  line L1480 (-25.1957, -17.7118) -> (-25.0625, -17.4964)
  line L1481 (-25.0625, -17.4964) -> (-24.931, -17.2934)
  line L1482 (-24.931, -17.2934) -> (-24.8029, -17.1047)
  line L1483 (-24.8029, -17.1047) -> (-24.6777, -16.928)
  line L1484 (-24.6777, -16.928) -> (-24.5555, -16.7632)
  line L1485 (-24.5555, -16.7632) -> (-24.4386, -16.6122)
  line L1486 (-24.4386, -16.6122) -> (-24.326, -16.4728)
  line L1487 (-24.326, -16.4728) -> (-24.0984, -16.2052)
  line L1488 (-24.0984, -16.2052) -> (-24.0735, -16.1655)
  line L1489 (-24.0735, -16.1655) -> (-24.0608, -16.1321)
  line L1490 (-24.0608, -16.1321) -> (-24.0599, -16.1055)
  line L1491 (-24.0599, -16.1055) -> (-24.0668, -16.0903)
  line L1492 (-24.0668, -16.0903) -> (-24.2795, -15.7673)
  line L1493 (-24.2795, -15.7673) -> (-24.488, -15.4416)
  line L1494 (-24.488, -15.4416) -> (-24.4991, -15.4291)
  line L1495 (-24.4991, -15.4291) -> (-24.5238, -15.4191)
  line L1496 (-24.5238, -15.4191) -> (-24.5595, -15.4172)
  line L1497 (-24.5595, -15.4172) -> (-24.6058, -15.4237)
  line L1498 (-24.6058, -15.4237) -> (-24.9429, -15.5228)
  line L1499 (-24.9429, -15.5228) -> (-25.1161, -15.569)
  line L1500 (-25.1161, -15.569) -> (-25.3015, -15.6144)
  line L1501 (-25.3015, -15.6144) -> (-25.5018, -15.6589)
  line L1502 (-25.5018, -15.6589) -> (-25.7142, -15.7015)
  line L1503 (-25.7142, -15.7015) -> (-25.9387, -15.7417)
  line L1504 (-25.9387, -15.7417) -> (-26.1776, -15.7793)
  line L1505 (-26.1776, -15.7793) -> (-26.4285, -15.8134)
  line L1506 (-26.4285, -15.8134) -> (-26.6482, -15.8389)
  arc A44 (-27.041, -15.1586) -> (-26.6482, -15.8389) centre (0, 0) ccw
  line L1507 (-27.041, -15.1586) -> (-26.9091, -14.9811)
  line L1508 (-26.9091, -14.9811) -> (-26.7541, -14.7808)
  line L1509 (-26.7541, -14.7808) -> (-26.602, -14.5927)
  line L1510 (-26.602, -14.5927) -> (-26.455, -14.4184)
  line L1511 (-26.455, -14.4184) -> (-26.312, -14.2558)
  line L1512 (-26.312, -14.2558) -> (-26.1732, -14.1046)
  line L1513 (-26.1732, -14.1046) -> (-26.0412, -13.9666)
  line L1514 (-26.0412, -13.9666) -> (-25.9146, -13.8398)
  line L1515 (-25.9146, -13.8398) -> (-25.6603, -13.5974)
  line L1516 (-25.6603, -13.5974) -> (-25.6314, -13.5605)
  line L1517 (-25.6314, -13.5605) -> (-25.6153, -13.5287)
  line L1518 (-25.6153, -13.5287) -> (-25.6116, -13.5023)
  line L1519 (-25.6116, -13.5023) -> (-25.6168, -13.4865)
  line L1520 (-25.6168, -13.4865) -> (-25.7946, -13.143)
  line L1521 (-25.7946, -13.143) -> (-25.968, -12.7973)
  line L1522 (-25.968, -12.7973) -> (-25.9777, -12.7837)
  line L1523 (-25.9777, -12.7837) -> (-26.0012, -12.7712)
  line L1524 (-26.0012, -12.7712) -> (-26.0365, -12.7656)
  line L1525 (-26.0365, -12.7656) -> (-26.0833, -12.7672)
  line L1526 (-26.0833, -12.7672) -> (-26.4288, -12.8305)
  line L1527 (-26.4288, -12.8305) -> (-26.6059, -12.8584)
  line L1528 (-26.6059, -12.8584) -> (-26.7951, -12.8841)
  line L1529 (-26.7951, -12.8841) -> (-26.9989, -12.9075)
  line L1530 (-26.9989, -12.9075) -> (-27.2145, -12.9276)
  line L1531 (-27.2145, -12.9276) -> (-27.442, -12.9441)
  line L1532 (-27.442, -12.9441) -> (-27.6836, -12.9565)
  line L1533 (-27.6836, -12.9565) -> (-27.9367, -12.9642)
  line L1534 (-27.9367, -12.9642) -> (-28.1579, -12.9667)
  arc A45 (-28.4774, -12.249) -> (-28.1579, -12.9667) centre (0, 0) ccw
  line L1535 (-28.4774, -12.249) -> (-28.3276, -12.0862)
  line L1536 (-28.3276, -12.0862) -> (-28.1525, -11.9033)
  line L1537 (-28.1525, -11.9033) -> (-27.9817, -11.7321)
  line L1538 (-27.9817, -11.7321) -> (-27.8172, -11.5741)
  line L1539 (-27.8172, -11.5741) -> (-27.6579, -11.4273)
  line L1540 (-27.6579, -11.4273) -> (-27.5042, -11.2915)
  line L1541 (-27.5042, -11.2915) -> (-27.3584, -11.1681)
  line L1542 (-27.3584, -11.1681) -> (-27.2193, -11.0551)
  line L1543 (-27.2193, -11.0551) -> (-26.941, -10.8407)
  line L1544 (-26.941, -10.8407) -> (-26.9085, -10.807)
  line L1545 (-26.9085, -10.807) -> (-26.8891, -10.777)
  line L1546 (-26.8891, -10.777) -> (-26.8826, -10.7512)
  line L1547 (-26.8826, -10.7512) -> (-26.8862, -10.7349)
  line L1548 (-26.8862, -10.7349) -> (-27.0272, -10.3748)
  line L1549 (-27.0272, -10.3748) -> (-27.1634, -10.0128)
  line L1550 (-27.1634, -10.0128) -> (-27.1717, -9.9983)
  line L1551 (-27.1717, -9.9983) -> (-27.1937, -9.9834)
  line L1552 (-27.1937, -9.9834) -> (-27.2282, -9.9741)
  line L1553 (-27.2282, -9.9741) -> (-27.2749, -9.9708)
  line L1554 (-27.2749, -9.9708) -> (-27.6252, -9.9977)
  line L1555 (-27.6252, -9.9977) -> (-27.8042, -10.0069)
  line L1556 (-27.8042, -10.0069) -> (-27.995, -10.0127)
  line L1557 (-27.995, -10.0127) -> (-28.2002, -10.0146)
  line L1558 (-28.2002, -10.0146) -> (-28.4168, -10.0121)
  line L1559 (-28.4168, -10.0121) -> (-28.6447, -10.0047)
  line L1560 (-28.6447, -10.0047) -> (-28.8863, -9.9918)
  line L1561 (-28.8863, -9.9918) -> (-29.1388, -9.973)
  line L1562 (-29.1388, -9.973) -> (-29.359, -9.9523)
  arc A46 (-29.6018, -9.2052) -> (-29.359, -9.9523) centre (0, 0) ccw
  line L1563 (-29.6018, -9.2052) -> (-29.4358, -9.059)
  line L1564 (-29.4358, -9.059) -> (-29.2425, -8.8954)
  line L1565 (-29.2425, -8.8954) -> (-29.0547, -8.7429)
  line L1566 (-29.0547, -8.7429) -> (-28.8746, -8.603)
  line L1567 (-28.8746, -8.603) -> (-28.7009, -8.4737)
  line L1568 (-28.7009, -8.4737) -> (-28.5338, -8.3547)
  line L1569 (-28.5338, -8.3547) -> (-28.3759, -8.2472)
  line L1570 (-28.3759, -8.2472) -> (-28.2257, -8.1494)
  line L1571 (-28.2257, -8.1494) -> (-27.9266, -7.9652)
  line L1572 (-27.9266, -7.9652) -> (-27.8907, -7.9351)
  line L1573 (-27.8907, -7.9351) -> (-27.8683, -7.9073)
  line L1574 (-27.8683, -7.9073) -> (-27.8592, -7.8823)
  line L1575 (-27.8592, -7.8823) -> (-27.861, -7.8657)
  line L1576 (-27.861, -7.8657) -> (-27.9636, -7.4928)
  line L1577 (-27.9636, -7.4928) -> (-28.0612, -7.1186)
  line L1578 (-28.0612, -7.1186) -> (-28.0679, -7.1033)
  line L1579 (-28.0679, -7.1033) -> (-28.0883, -7.0862)
  line L1580 (-28.0883, -7.0862) -> (-28.1216, -7.0733)
  line L1581 (-28.1216, -7.0733) -> (-28.1677, -7.0652)
  line L1582 (-28.1677, -7.0652) -> (-28.5189, -7.0553)
  line L1583 (-28.5189, -7.0553) -> (-28.6979, -7.0457)
  line L1584 (-28.6979, -7.0457) -> (-28.8883, -7.0315)
  line L1585 (-28.8883, -7.0315) -> (-29.0926, -7.012)
  line L1586 (-29.0926, -7.012) -> (-29.3077, -6.9869)
  line L1587 (-29.3077, -6.9869) -> (-29.5336, -6.9557)
  line L1588 (-29.5336, -6.9557) -> (-29.7725, -6.9177)
  line L1589 (-29.7725, -6.9177) -> (-30.0216, -6.8726)
  line L1590 (-30.0216, -6.8726) -> (-30.2385, -6.829)
  arc A47 (-30.4018, -6.0605) -> (-30.2385, -6.829) centre (0, 0) ccw
  line L1591 (-30.4018, -6.0605) -> (-30.2214, -5.9325)
  line L1592 (-30.2214, -5.9325) -> (-30.0122, -5.79)
  line L1593 (-30.0122, -5.79) -> (-29.8094, -5.658)
  line L1594 (-29.8094, -5.658) -> (-29.6157, -5.5376)
  line L1595 (-29.6157, -5.5376) -> (-29.4294, -5.4272)
  line L1596 (-29.4294, -5.4272) -> (-29.2508, -5.3263)
  line L1597 (-29.2508, -5.3263) -> (-29.0826, -5.2359)
  line L1598 (-29.0826, -5.2359) -> (-28.9229, -5.1544)
  line L1599 (-28.9229, -5.1544) -> (-28.6062, -5.0025)
  line L1600 (-28.6062, -5.0025) -> (-28.5674, -4.9763)
  line L1601 (-28.5674, -4.9763) -> (-28.5421, -4.951)
  line L1602 (-28.5421, -4.951) -> (-28.5305, -4.927)
  line L1603 (-28.5305, -4.927) -> (-28.5306, -4.9104)
  line L1604 (-28.5306, -4.9104) -> (-28.5936, -4.5288)
  line L1605 (-28.5936, -4.5288) -> (-28.6516, -4.1464)
  line L1606 (-28.6516, -4.1464) -> (-28.6567, -4.1305)
  line L1607 (-28.6567, -4.1305) -> (-28.6751, -4.1114)
  line L1608 (-28.6751, -4.1114) -> (-28.7069, -4.0951)
  line L1609 (-28.7069, -4.0951) -> (-28.7519, -4.0822)
  line L1610 (-28.7519, -4.0822) -> (-29.1001, -4.0356)
  line L1611 (-29.1001, -4.0356) -> (-29.2771, -4.0074)
  line L1612 (-29.2771, -4.0074) -> (-29.465, -3.9734)
  line L1613 (-29.465, -3.9734) -> (-29.6661, -3.9326)
  line L1614 (-29.6661, -3.9326) -> (-29.8774, -3.8852)
  line L1615 (-29.8774, -3.8852) -> (-30.0989, -3.8305)
  line L1616 (-30.0989, -3.8305) -> (-30.3325, -3.7677)
  line L1617 (-30.3325, -3.7677) -> (-30.5755, -3.6968)
  line L1618 (-30.5755, -3.6968) -> (-30.7866, -3.6308)
  arc A48 (-30.8688, -2.8495) -> (-30.7866, -3.6308) centre (0, 0) ccw
  line L1619 (-30.8688, -2.8495) -> (-30.676, -2.741)
  line L1620 (-30.676, -2.741) -> (-30.453, -2.6211)
  line L1621 (-30.453, -2.6211) -> (-30.2376, -2.5111)
  line L1622 (-30.2376, -2.5111) -> (-30.0323, -2.4116)
  line L1623 (-30.0323, -2.4116) -> (-29.8355, -2.3213)
  line L1624 (-29.8355, -2.3213) -> (-29.6473, -2.2396)
  line L1625 (-29.6473, -2.2396) -> (-29.4705, -2.1673)
  line L1626 (-29.4705, -2.1673) -> (-29.3033, -2.1029)
  line L1627 (-29.3033, -2.1029) -> (-28.9724, -1.9849)
  line L1628 (-28.9724, -1.9849) -> (-28.931, -1.9629)
  line L1629 (-28.931, -1.9629) -> (-28.9033, -1.9404)
  line L1630 (-28.9033, -1.9404) -> (-28.8892, -1.9178)
  line L1631 (-28.8892, -1.9178) -> (-28.8876, -1.9012)
  line L1632 (-28.8876, -1.9012) -> (-28.9103, -1.5151)
  line L1633 (-28.9103, -1.5151) -> (-28.9281, -1.1288)
  line L1634 (-28.9281, -1.1288) -> (-28.9314, -1.1124)
  line L1635 (-28.9314, -1.1124) -> (-28.9478, -1.0915)
  line L1636 (-28.9478, -1.0915) -> (-28.9777, -1.0719)
  line L1637 (-28.9777, -1.0719) -> (-29.0211, -1.0544)
  line L1638 (-29.0211, -1.0544) -> (-29.3626, -0.9717)
  line L1639 (-29.3626, -0.9717) -> (-29.5356, -0.9251)
  line L1640 (-29.5356, -0.9251) -> (-29.719, -0.8717)
  line L1641 (-29.719, -0.8717) -> (-29.9147, -0.8101)
  line L1642 (-29.9147, -0.8101) -> (-30.1199, -0.7408)
  line L1643 (-30.1199, -0.7408) -> (-30.3344, -0.6634)
  line L1644 (-30.3344, -0.6634) -> (-30.5601, -0.5765)
  line L1645 (-30.5601, -0.5765) -> (-30.7945, -0.4805)
  line L1646 (-30.7945, -0.4805) -> (-30.9975, -0.3928)
  arc A49 (-30.9975, 0.3928) -> (-30.9975, -0.3928) centre (0, 0) ccw
  line L1647 (-30.9975, 0.3928) -> (-30.7945, 0.4805)
  line L1648 (-30.7945, 0.4805) -> (-30.5601, 0.5765)
  line L1649 (-30.5601, 0.5765) -> (-30.3344, 0.6634)
  line L1650 (-30.3344, 0.6634) -> (-30.1199, 0.7408)
  line L1651 (-30.1199, 0.7408) -> (-29.9147, 0.8101)
  line L1652 (-29.9147, 0.8101) -> (-29.719, 0.8717)
  line L1653 (-29.719, 0.8717) -> (-29.5356, 0.9251)
  line L1654 (-29.5356, 0.9251) -> (-29.3626, 0.9717)
  line L1655 (-29.3626, 0.9717) -> (-29.0211, 1.0544)
  line L1656 (-29.0211, 1.0544) -> (-28.9777, 1.0719)
  line L1657 (-28.9777, 1.0719) -> (-28.9478, 1.0915)
  line L1658 (-28.9478, 1.0915) -> (-28.9314, 1.1124)
  line L1659 (-28.9314, 1.1124) -> (-28.9281, 1.1288)
  line L1660 (-28.9281, 1.1288) -> (-28.9103, 1.5151)
  line L1661 (-28.9103, 1.5151) -> (-28.8876, 1.9012)
  line L1662 (-28.8876, 1.9012) -> (-28.8892, 1.9178)
  line L1663 (-28.8892, 1.9178) -> (-28.9033, 1.9404)
  line L1664 (-28.9033, 1.9404) -> (-28.931, 1.9629)
  line L1665 (-28.931, 1.9629) -> (-28.9724, 1.9849)
  line L1666 (-28.9724, 1.9849) -> (-29.3033, 2.1029)
  line L1667 (-29.3033, 2.1029) -> (-29.4705, 2.1673)
  line L1668 (-29.4705, 2.1673) -> (-29.6473, 2.2396)
  line L1669 (-29.6473, 2.2396) -> (-29.8355, 2.3213)
  line L1670 (-29.8355, 2.3213) -> (-30.0323, 2.4116)
  line L1671 (-30.0323, 2.4116) -> (-30.2376, 2.5111)
  line L1672 (-30.2376, 2.5111) -> (-30.453, 2.6211)
  line L1673 (-30.453, 2.6211) -> (-30.676, 2.741)
  line L1674 (-30.676, 2.741) -> (-30.8688, 2.8495)
  arc A50 (-30.7866, 3.6308) -> (-30.8688, 2.8495) centre (0, 0) ccw
  line L1675 (-30.7866, 3.6308) -> (-30.5755, 3.6968)
  line L1676 (-30.5755, 3.6968) -> (-30.3325, 3.7677)
  line L1677 (-30.3325, 3.7677) -> (-30.0989, 3.8305)
  line L1678 (-30.0989, 3.8305) -> (-29.8774, 3.8852)
  line L1679 (-29.8774, 3.8852) -> (-29.6661, 3.9326)
  line L1680 (-29.6661, 3.9326) -> (-29.465, 3.9734)
  line L1681 (-29.465, 3.9734) -> (-29.2771, 4.0074)
  line L1682 (-29.2771, 4.0074) -> (-29.1001, 4.0356)
  line L1683 (-29.1001, 4.0356) -> (-28.7519, 4.0822)
  line L1684 (-28.7519, 4.0822) -> (-28.7069, 4.0951)
  line L1685 (-28.7069, 4.0951) -> (-28.6751, 4.1114)
  line L1686 (-28.6751, 4.1114) -> (-28.6567, 4.1305)
  line L1687 (-28.6567, 4.1305) -> (-28.6516, 4.1464)
  line L1688 (-28.6516, 4.1464) -> (-28.5936, 4.5288)
  line L1689 (-28.5936, 4.5288) -> (-28.5306, 4.9104)
  line L1690 (-28.5306, 4.9104) -> (-28.5305, 4.927)
  line L1691 (-28.5305, 4.927) -> (-28.5421, 4.951)
  line L1692 (-28.5421, 4.951) -> (-28.5674, 4.9763)
  line L1693 (-28.5674, 4.9763) -> (-28.6062, 5.0025)
  line L1694 (-28.6062, 5.0025) -> (-28.9229, 5.1544)
  line L1695 (-28.9229, 5.1544) -> (-29.0826, 5.2359)
  line L1696 (-29.0826, 5.2359) -> (-29.2508, 5.3263)
  line L1697 (-29.2508, 5.3263) -> (-29.4294, 5.4272)
  line L1698 (-29.4294, 5.4272) -> (-29.6157, 5.5376)
  line L1699 (-29.6157, 5.5376) -> (-29.8094, 5.658)
  line L1700 (-29.8094, 5.658) -> (-30.0122, 5.79)
  line L1701 (-30.0122, 5.79) -> (-30.2214, 5.9325)
  line L1702 (-30.2214, 5.9325) -> (-30.4018, 6.0605)
  arc A51 (-30.2385, 6.829) -> (-30.4018, 6.0605) centre (0, 0) ccw
  line L1703 (-30.2385, 6.829) -> (-30.0216, 6.8726)
  line L1704 (-30.0216, 6.8726) -> (-29.7725, 6.9177)
  line L1705 (-29.7725, 6.9177) -> (-29.5336, 6.9557)
  line L1706 (-29.5336, 6.9557) -> (-29.3077, 6.9869)
  line L1707 (-29.3077, 6.9869) -> (-29.0926, 7.012)
  line L1708 (-29.0926, 7.012) -> (-28.8883, 7.0315)
  line L1709 (-28.8883, 7.0315) -> (-28.6979, 7.0457)
  line L1710 (-28.6979, 7.0457) -> (-28.5189, 7.0553)
  line L1711 (-28.5189, 7.0553) -> (-28.1677, 7.0652)
  line L1712 (-28.1677, 7.0652) -> (-28.1216, 7.0733)
  line L1713 (-28.1216, 7.0733) -> (-28.0883, 7.0862)
  line L1714 (-28.0883, 7.0862) -> (-28.0679, 7.1033)
  line L1715 (-28.0679, 7.1033) -> (-28.0612, 7.1186)
  line L1716 (-28.0612, 7.1186) -> (-27.9636, 7.4928)
  line L1717 (-27.9636, 7.4928) -> (-27.861, 7.8657)
  line L1718 (-27.861, 7.8657) -> (-27.8592, 7.8823)
  line L1719 (-27.8592, 7.8823) -> (-27.8683, 7.9073)
  line L1720 (-27.8683, 7.9073) -> (-27.8907, 7.9351)
  line L1721 (-27.8907, 7.9351) -> (-27.9266, 7.9652)
  line L1722 (-27.9266, 7.9652) -> (-28.2257, 8.1494)
  line L1723 (-28.2257, 8.1494) -> (-28.3759, 8.2472)
  line L1724 (-28.3759, 8.2472) -> (-28.5338, 8.3547)
  line L1725 (-28.5338, 8.3547) -> (-28.7009, 8.4737)
  line L1726 (-28.7009, 8.4737) -> (-28.8746, 8.603)
  line L1727 (-28.8746, 8.603) -> (-29.0547, 8.7429)
  line L1728 (-29.0547, 8.7429) -> (-29.2425, 8.8954)
  line L1729 (-29.2425, 8.8954) -> (-29.4358, 9.059)
  line L1730 (-29.4358, 9.059) -> (-29.6018, 9.2052)
  arc A52 (-29.359, 9.9523) -> (-29.6018, 9.2052) centre (0, 0) ccw
  line L1731 (-29.359, 9.9523) -> (-29.1388, 9.973)
  line L1732 (-29.1388, 9.973) -> (-28.8863, 9.9918)
  line L1733 (-28.8863, 9.9918) -> (-28.6447, 10.0047)
  line L1734 (-28.6447, 10.0047) -> (-28.4168, 10.0121)
  line L1735 (-28.4168, 10.0121) -> (-28.2002, 10.0146)
  line L1736 (-28.2002, 10.0146) -> (-27.995, 10.0127)
  line L1737 (-27.995, 10.0127) -> (-27.8042, 10.0069)
  line L1738 (-27.8042, 10.0069) -> (-27.6252, 9.9977)
  line L1739 (-27.6252, 9.9977) -> (-27.2749, 9.9708)
  line L1740 (-27.2749, 9.9708) -> (-27.2282, 9.9741)
  line L1741 (-27.2282, 9.9741) -> (-27.1937, 9.9834)
  line L1742 (-27.1937, 9.9834) -> (-27.1717, 9.9983)
  line L1743 (-27.1717, 9.9983) -> (-27.1634, 10.0128)
  line L1744 (-27.1634, 10.0128) -> (-27.0272, 10.3748)
  line L1745 (-27.0272, 10.3748) -> (-26.8862, 10.7349)
  line L1746 (-26.8862, 10.7349) -> (-26.8826, 10.7512)
  line L1747 (-26.8826, 10.7512) -> (-26.8891, 10.777)
  line L1748 (-26.8891, 10.777) -> (-26.9085, 10.807)
  line L1749 (-26.9085, 10.807) -> (-26.941, 10.8407)
  line L1750 (-26.941, 10.8407) -> (-27.2193, 11.0551)
  line L1751 (-27.2193, 11.0551) -> (-27.3584, 11.1681)
  line L1752 (-27.3584, 11.1681) -> (-27.5042, 11.2915)
  line L1753 (-27.5042, 11.2915) -> (-27.6579, 11.4273)
  line L1754 (-27.6579, 11.4273) -> (-27.8172, 11.5741)
  line L1755 (-27.8172, 11.5741) -> (-27.9817, 11.7321)
  line L1756 (-27.9817, 11.7321) -> (-28.1525, 11.9033)
  line L1757 (-28.1525, 11.9033) -> (-28.3276, 12.0862)
  line L1758 (-28.3276, 12.0862) -> (-28.4774, 12.249)
  arc A53 (-28.1579, 12.9667) -> (-28.4774, 12.249) centre (0, 0) ccw
  line L1759 (-28.1579, 12.9667) -> (-27.9367, 12.9642)
  line L1760 (-27.9367, 12.9642) -> (-27.6836, 12.9565)
  line L1761 (-27.6836, 12.9565) -> (-27.442, 12.9441)
  line L1762 (-27.442, 12.9441) -> (-27.2145, 12.9276)
  line L1763 (-27.2145, 12.9276) -> (-26.9989, 12.9075)
  line L1764 (-26.9989, 12.9075) -> (-26.7951, 12.8841)
  line L1765 (-26.7951, 12.8841) -> (-26.6059, 12.8584)
  line L1766 (-26.6059, 12.8584) -> (-26.4288, 12.8305)
  line L1767 (-26.4288, 12.8305) -> (-26.0833, 12.7672)
  line L1768 (-26.0833, 12.7672) -> (-26.0365, 12.7656)
  line L1769 (-26.0365, 12.7656) -> (-26.0012, 12.7712)
  line L1770 (-26.0012, 12.7712) -> (-25.9777, 12.7837)
  line L1771 (-25.9777, 12.7837) -> (-25.968, 12.7973)
  line L1772 (-25.968, 12.7973) -> (-25.7946, 13.143)
  line L1773 (-25.7946, 13.143) -> (-25.6168, 13.4865)
  line L1774 (-25.6168, 13.4865) -> (-25.6116, 13.5023)
  line L1775 (-25.6116, 13.5023) -> (-25.6153, 13.5287)
  line L1776 (-25.6153, 13.5287) -> (-25.6314, 13.5605)
  line L1777 (-25.6314, 13.5605) -> (-25.6603, 13.5974)
  line L1778 (-25.6603, 13.5974) -> (-25.9146, 13.8398)
  line L1779 (-25.9146, 13.8398) -> (-26.0412, 13.9666)
  line L1780 (-26.0412, 13.9666) -> (-26.1732, 14.1046)
  line L1781 (-26.1732, 14.1046) -> (-26.312, 14.2558)
  line L1782 (-26.312, 14.2558) -> (-26.455, 14.4184)